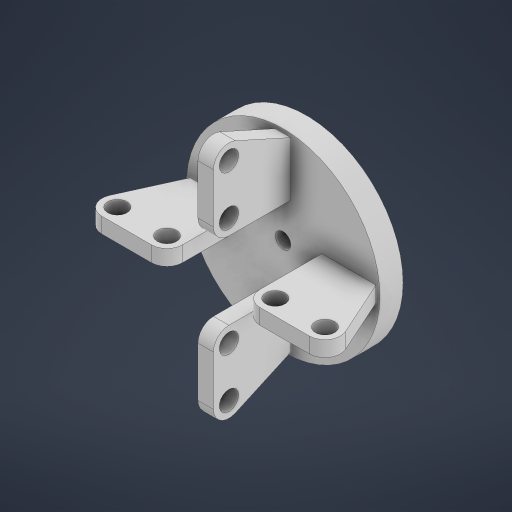
# Autodesk Inventor part: Base
Saved by Autodesk Inventor 2023 (Build 270158000, 158)
## iProperties
Created: 2023-04-12
Part Number: Base
Material: Generic
Document SubType Name: Modeling
Designer: vatdu
Density: 1 g/cm^3
Appearance: Default
Author: vatdu
Autodesk Inventor part; units mm, degrees
ref_plane "YZ Plane" through (0, 0, 0) normal (1, 0, 0) x (0, 1, 0)
ref_plane "XZ Plane" through (0, 0, 0) normal (0, 1, 0) x (-1, 0, 0)
ref_plane "XY Plane" through (0, 0, 0) normal (0, 0, 1) x (1, 0, 0)
sketch "Sketch1" plane through (0, 0, 0) normal (0, 0, 1) x (1, 0, 0)
  circle A0 centre (0, 0) radius 12.5
  dimension "d0" = 25
  constraints: 1 centre point, 1 coincident
  measures "d0" diameter of A0
extrude "Extrusion1" add sketch "Sketch1" along normal blind 3
sketch "Sketch2" plane through (0, 0, 3) normal (0, 0, 1) x (1, 0, 0)
  circle A0 centre (0, 0) radius 1
  dimension "d3" = 2
  constraints: 1 centre point, 1 coincident
  measures "d3" diameter of A0
extrude "Extrusion2" cut sketch "Sketch2" against normal blind 3
sketch "Sketch3" plane through (0, 0, 3) normal (0, 0, 1) x (1, 0, 0)
  circle A0 centre (0, 0) radius 12.5 projected
  line L0 (1, 5) -> (-1, 5)
  line L1 (-1, 5) -> (-1, 16.5124)
  line L2 (-1, 16.5124) -> (1, 16.5124)
  line L3 (1, 16.5124) -> (1, 5)
  line L4 (-5, -1) -> (-16.5124, -1)
  line L5 (-16.5124, -1) -> (-16.5124, 1)
  line L6 (-16.5124, 1) -> (-5, 1)
  line L7 (-5, 1) -> (-5, -1)
  line L8 (1, -5) -> (1, -16.5124)
  line L9 (1, -16.5124) -> (-1, -16.5124)
  line L10 (-1, -16.5124) -> (-1, -5)
  line L11 (-1, -5) -> (1, -5)
  line L12 (5, 1) -> (16.5124, 1)
  line L13 (16.5124, 1) -> (16.5124, -1)
  line L14 (16.5124, -1) -> (5, -1)
  line L15 (5, -1) -> (5, 1)
  point P0 (-1, -12.4599)
  point P1 (1, -12.4599)
  point P2 (12.4599, -1)
  point P3 (12.4599, 1)
  point P4 (1, 12.4599)
  point P5 (-1, 12.4599)
  point P6 (-12.4599, 1)
  point P7 (-12.4599, -1)
  dimension "d8" = 2
  dimension "d11" = 360
  constraints: 32 end point, 2 parallel, 1 horizontal, 1 perpendicular, 33 other
  measures "d8" distance of L1.end L2.end
extrude "Extrusion3" add sketch "Sketch3" along normal blind 10 contours A0 L14 L15 L12 | A0 L12 L13 L14 | L3 L0 L1 A0 | A0 L1 L2 L3 | L8 L9 L10 A0 | A0 L10 L11 L8 | L6 L7 L4 A0 | A0 L4 L5 L6
sketch "Sketch5" plane through (1, 12.4599, 3) normal (1, 0, 0) x (0, 0, -1)
  line L0 (0, -7.4599) -> (-10, -7.4599) projected
  line L1 (0, 0) -> (0, 4.0525) projected
  line L2 (-10, -7.4599) -> (0, -7.4599)
  line L3 (0, -7.4599) -> (0, 4.0525)
  line L4 (0, 4.0525) -> (-10, 4.0525)
  line L5 (-10, 4.0525) -> (-10, -7.4599)
  line L6 (0, -7.4599) -> (0, -0.4599)
  line L7 (0, 0) -> (0, -11.4599) projected
  line L8 (-10, -7.4599) -> (-10, 4.0525) projected
  line L9 (0, -0.4599) -> (-10, 4.0525)
  point P0 (3, -12.4599)
  point P1 (0, -0.4599)
  dimension "d26" = 7
  constraints: 12 end point, 2 parallel, 1 horizontal, 1 perpendicular, 1 point on line
  measures "d26" distance of L2.end L6.end
extrude "Extrusion5" cut sketch "Sketch5" against normal blind 10 contours L9 L4 L1 L3
pattern_circular "Circular Pattern3" count 4 over 360 about axis through (0, 0, 3) along (0, 0, -1) of "Extrusion5"
fillet "Fillet2" radius 2 8 edges at (0, 16.5124, 13) (0, 5, 13) (-5, 0, 13) (-16.5124, 0, 13) (0, -5, 13) (0, -16.5124, 13) (5, 0, 13) (16.5124, 0, 13)
sketch "Sketch6" plane through (1, -12, 3) normal (1, 0, 0) x (0, 0, -1)
  arc A0 (-10, -1.4157) -> (-7.1774, -3.2387) centre (-8, -1.4157) ccw projected
  circle A1 centre (-8, -1.4157) radius 1.25
  arc A2 (-8, 7) -> (-10, 5) centre (-8, 5) ccw projected
  circle A3 centre (-8, 5) radius 1.25
  point P0 (3, 12)
  dimension "d33" = 2.5
  dimension "d34" = 2.5
  constraints: 2 centre point, 2 coincident
  measures "d33" diameter of A1
  measures "d34" diameter of A3
extrude "Extrusion6" cut sketch "Sketch6" against normal blind 10
pattern_circular "Circular Pattern4" count 4 over 360 about axis through (0, 0, 3) along (0, 0, -1) of "Extrusion6"
body "Solid1"
